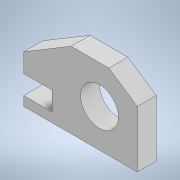
# Autodesk Inventor part: Assignment 4.1 - Inclined Support
Saved by Autodesk Inventor 2022 (Build 260153000, 153)
## iProperties
Created: 2021-05-24
Part Number: Assignment 4.1 - Inclined Support
Material: Generic
Document SubType Name: Modeling
Designer: Aaron
Density: 1 g/cm^3
Appearance: Default
Author: Aaron
Autodesk Inventor part; units mm, degrees
ref_plane "YZ Plane" through (0, 0, 0) normal (1, 0, 0) x (0, 1, 0)
ref_plane "XZ Plane" through (0, 0, 0) normal (0, 1, 0) x (-1, 0, 0)
ref_plane "XY Plane" through (0, 0, 0) normal (0, 0, 1) x (1, 0, 0)
sketch "Sketch1" plane through (0, 0, 0) normal (0, 0, 1) x (1, 0, 0)
  line L0 (0, 0) -> (76.2, 0)
  line L1 (76.2, 0) -> (76.2, 38.1)
  line L2 (57.15, 50.8) -> (76.2, 38.1)
  line L3 (57.15, 50.8) -> (31.75, 50.8)
  line L4 (0, 0) -> (0, 6.35)
  line L5 (0, 6.35) -> (19.05, 6.35)
  line L6 (19.05, 6.35) -> (19.05, 19.05)
  line L7 (19.05, 19.05) -> (0, 19.05)
  line L8 (0, 19.05) -> (0, 31.75)
  line L9 (0, 31.75) -> (31.75, 50.8)
  circle A0 centre (50.8, 25.4) radius 12.7
  dimension "d1" = 76.2
  dimension "d2" = 38.1
  dimension "d5" = 25.4
  dimension "d6" = 6.35
  dimension "d7" = 19.05
  dimension "d8" = 12.7
  dimension "d9" = 19.05
  dimension "d10" = 12.7
  dimension "d13" = 25.4
  constraints: 20 end point, 3 perpendicular, 2 horizontal, 2 point on line, 1 centre point, 1 vertical
  measures "d1" distance of L0.start L0.end
  measures "d2" distance of L0.end L1.end
  measures "d5" distance of L2.start L3.end
  measures "d6" distance of L0.start L4.end
  measures "d7" distance of L4.end L5.end
  measures "d8" distance of L5.end L6.end
  measures "d9" distance of L6.end L7.end
  measures "d10" distance of L7.end L8.end
  measures "d13" diameter of A0
extrude "Extrusion1" add sketch "Sketch1" along normal blind 12.7
body "Solid1"
